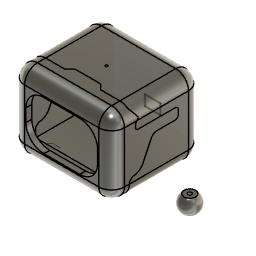
Astrobot clock outside v14 (Autodesk Fusion 360 design; units mm, degrees)
Autodesk Fusion 360 part; units mm, degrees
sketch "Sketch2" plane through (0, 0, 0) normal (0, 0, 1) x (1, 0, 0)
  line L0 (39, 35) -> (-39, 35)
  line L1 (-39, 35) -> (-39, -35)
  line L2 (-39, -35) -> (39, -35)
  line L3 (39, -35) -> (39, 35)
  line L4 (39, 35) -> (-39, -35) construction
  line L5 (-39, 35) -> (39, -35) construction
  dimension "d5" = 78
  dimension "d6" = 70
  constraint horizontal L0
  constraint perpendicular L0 L1
  constraint parallel L0 L2
  constraint parallel L1 L3
  constraint coincident L4 origin
  constraint coincident L5 origin
  measures "d5" distance of L1.end L2.end
  measures "d6" distance of L0.end L1.end
extrude "Extrude1" add sketch "Sketch2" along normal blind 60 makes body 1
fillet "Fillet2" radius 10 10 edges at (-39, 35, 30) (39, -35, 30) (0, 35, 0) (0, -35, 60) (39, 35, 30) (39, 0, 0) (-39, -35, 30) (-39, 0, 60) (-39, 0, 0) (39, 0, 60) 5 faces at (39, -11.6667, 20) (-39, 11.6667, 20) (-13, -35, 40) (13, -11.6667, 0) (13, 35, 40) on bodies 1
sketch "Sketch19" plane through (0, -35, 0) normal (0, -1, 0) x (1, 0, 0)
  line L0 (-29, 10) -> (29, 10)
  line L1 (29, 10) -> (29, 50)
  line L2 (29, 50) -> (-29, 50)
  line L3 (-29, 50) -> (-29, 10)
  line L4 (-14, 50) -> (14, 50)
  line L5 (29, 35) -> (29, 25)
  line L6 (14, 10) -> (-14, 10)
  line L7 (-29, 25) -> (-29, 35)
  arc A0 (-14, 50) -> (-29, 35) centre (-14, 35) ccw
  arc A1 (-29, 25) -> (-14, 10) centre (-14, 25) ccw
  arc A2 (14, 10) -> (29, 25) centre (14, 25) ccw
  arc A3 (29, 35) -> (14, 50) centre (14, 35) ccw
  arc A4 (28, 35) -> (14, 49) centre (14, 35) ccw
  line L8 (-14, 49) -> (14, 49)
  arc A5 (-14, 49) -> (-28, 35) centre (-14, 35) ccw
  line L9 (-28, 25) -> (-28, 35)
  arc A6 (-28, 25) -> (-14, 11) centre (-14, 25) ccw
  line L10 (14, 11) -> (-14, 11)
  arc A7 (14, 11) -> (28, 25) centre (14, 25) ccw
  line L11 (28, 35) -> (28, 25)
  dimension "d109" = 15
  dimension "d110" = 1
  constraint horizontal L4
  constraint vertical L5
  constraint horizontal L6
  constraint vertical L7
  constraint tangent L4 A0
  constraint tangent L7 A0
  constraint tangent L6 A1
  constraint tangent L7 A1
  constraint equal A0 A1
  constraint tangent L5 A2
  constraint tangent L6 A2
  constraint equal A0 A2
  constraint tangent L4 A3
  constraint tangent L5 A3
  constraint equal A0 A3
  measures "d109" radius of A0
extrude "Extrude15" cut sketch "Sketch19" against normal blind 42 contours A4 L8 A5 L9 A6 L10 A7 L11 bodies 1
sketch "Sketch3" plane through (39, 0, 0) normal (1, 0, 0) x (0, 1, 0)
  line L0 (-25, 10) -> (25, 10)
  line L1 (25, 10) -> (25, 50)
  line L2 (25, 50) -> (-25, 50)
  line L3 (-25, 50) -> (-25, 10)
  line L4 (-18.6068, 75) -> (-18.6068, 57.9889)
  line L5 (-18.6068, 57.9889) -> (-13.9508, 51.5222)
  line L6 (-13.9508, 51.5222) -> (-16.313, 48.3417)
  line L7 (-15.1681, 43.7622) -> (14.5844, 43.7622)
  line L8 (17.1014, 43.7622) -> (17.1014, 42.6668)
  line L9 (14.5617, 35.4315) -> (0.4578, 35.4315)
  line L10 (-4.0631, 32.5672) -> (-10, 20)
  arc A0 (-18.7241, 13.8606) -> (-10, 20) centre (-18.605, 22.9596) ccw
  line L11 (-21.0542, 11.5608) -> (-21.0542, 0)
  line L12 (-21.0542, 0) -> (-21.0542, -15)
  line L13 (-21.0542, -15) -> (-21.0542, -16.3731)
  spline S0 degree 5 poles (17.1014, 43.7622) (17.189, 43.7622) (17.3347, 43.7478) (17.4648, 43.6829) (17.4892, 43.5233) (17.3771, 43.252) (17.2511, 43.0139) (17.1681, 42.8378) (17.1221, 42.7233) (17.1014, 42.6668) knots 0 0 0 0 0 0 0.2 0.4 0.6 0.8 1 1 1 1 1 1
  line L14 (17.0843, 41.2452) -> (17.0617, 37.9145)
  arc A1 (17.0843, 41.2452) -> (14.5844, 43.7622) centre (14.5844, 41.2622) ccw
  arc A2 (14.5617, 35.4315) -> (17.0617, 37.9145) centre (14.5617, 37.9315) ccw
  arc A3 (0.4578, 35.4315) -> (-4.0631, 32.5672) centre (0.4578, 30.4315) ccw
  line L15 (-16.313, 48.3417) -> (-16.313, 44.9071)
  line L16 (-16.313, 44.9071) -> (-15.1681, 43.7622)
  line L17 (-18.7241, 13.8606) -> (-21.0542, 11.5608)
  point P0 (-16.313, 43.7622)
  dimension "d113" = 2.5
  dimension "d114" = 5
  dimension "d116" = 1.1449
  dimension "d117" = 1.1449
  constraint vertical L4
  constraint horizontal L7
  constraint perpendicular L7 L8
  constraint parallel L7 L9
  constraint perpendicular L0 L11
  constraint perpendicular L0 L12
  constraint perpendicular L0 L13
  constraint coincident L8.start L7
  constraint coincident L8.start L14
  constraint tangent L7 A1
  constraint tangent L14 A1
  constraint tangent L14 A2
  constraint tangent L9 A2
  constraint equal A1 A2
  constraint tangent L9 A3
  constraint tangent L10 A3
  constraint perpendicular L7 L15
  constraint coincident L15 P0
  constraint coincident L7 P0
  measures "d113" radius of A1
  measures "d114" radius of A3
  measures "d116" distance of L15.end P0
  measures "d117" distance of L7.start P0
split "Split1" by curves path "Sketch3" along L4 L5 L6 L15 L16 L7 A1 L14 A2 L9 A3 L10 A0 L17 L11 L12 L13 bodies 1 makes body 2 at (-9.6667, 9.6486, 0)
sketch "Sketch6" plane through (0, 0, 0) normal (0, 0, 1) x (1, 0, 0)
  line L0 (34, 30) -> (-34, 30)
  line L1 (-34, 30) -> (-34, -30)
  line L2 (-34, -30) -> (34, -30)
  line L3 (34, -30) -> (34, 30)
  line L4 (34, 30) -> (-34, -30) construction
  line L5 (-34, 30) -> (34, -30) construction
  dimension "d13" = 68
  dimension "d14" = 60
  constraint horizontal L0
  constraint perpendicular L0 L1
  constraint parallel L0 L2
  constraint parallel L1 L3
  constraint coincident L4 origin
  constraint coincident L5 origin
  measures "d13" distance of L1.end L2.end
  measures "d14" distance of L0.end L1.end
extrude "Extrude3" add sketch "Sketch6" along normal blind 50 separate body makes body 3
move_face "OffsetFaces1" offset 0.4 6 faces at (-11.3333, -30, 16.6667) (-34, 10, 33.3333) (-11.3333, 10, 50) (-11.3333, 10, 0) (34, -10, 33.3333) (11.3333, 30, 16.6667) on bodies 3
move_body "Move1" bodies 3 to x (1, 0, 0) y (0, 1, 0) z (0, 0, 1) at (0, 0, 5)
sketch "Sketch9" plane through (0, 0, 60) normal (0, 0, 1) x (-1, 0, 0)
  line L0 (-29, -25) -> (29, -25)
  line L1 (29, -25) -> (29, 18.6068)
  circle A0 centre (0, 0) radius 0.9
  line L2 (-29, 18.6068) -> (-29, -25)
  line L3 (29, 18.6068) -> (-29, 18.6068)
  dimension "d17" = 1.8
  constraint coincident A0.centre origin
  measures "d17" diameter of A0
extrude "Extrude4" cut sketch "Sketch9" against normal blind 3 contours A0 bodies 2
combine "Combine18" operation cut target body 2 tool bodies 3 keep tools
combine "Combine20" operation cut target body 1 tool bodies 3 keep tools
sketch "Sketch15" plane through (0, -18.6068, 0) normal (0, 1, 0) x (-1, 0, 0)
  arc A0 (-29, 60) -> (-35.0148, 57.9889) centre (-29, 50) ccw
  line L0 (-35.0148, 57.9889) -> (35.0148, 57.9889)
  arc A1 (35.0148, 57.9889) -> (29, 60) centre (29, 50) ccw
  line L1 (29, 60) -> (-29, 60)
  line L2 (10, 55.9778) -> (-10, 55.9778)
  line L3 (-10, 55.9778) -> (-10, 60)
  line L4 (-10, 60) -> (10, 60)
  line L5 (10, 60) -> (10, 55.9778)
  line L6 (10, 55.9778) -> (-10, 60) construction
  line L7 (-10, 55.9778) -> (10, 60) construction
  point P0 (0, 57.9889)
  constraint horizontal L2
  constraint perpendicular L2 L3
  constraint parallel L2 L4
  constraint parallel L3 L5
  constraint coincident L6 P0
  constraint coincident L7 P0
  constraint midpoint L0 P0
  constraint coincident L1 L3.end
extrude "Extrude11" add sketch "Sketch15" along normal blind 4 contours L0 L1 L3 L4 L5 bodies 1
chamfer "Chamfer1" distance 4 angle 45 2 edges at (10, -18.6068, 58.9944) (-10, -18.6068, 58.9944) on bodies 1
sketch "Sketch16" plane through (0, -21.0542, 0) normal (0, 1, 0) x (-1, 0, 0)
  line L0 (34.4, 11.5608) -> (34.4, 4.6)
  line L1 (34.4, 4.6) -> (-34.4, 4.6)
  line L2 (-34.4, 4.6) -> (-34.4, 11.5608)
  line L3 (-39, 11.5608) -> (-39, 10)
  arc A0 (-39, 10) -> (-29, 0) centre (-29, 10) ccw
  line L4 (-29, 0) -> (29, 0)
  arc A1 (29, 0) -> (39, 10) centre (29, 10) ccw
  line L5 (39, 10) -> (39, 11.5608)
  line L6 (-24, 4) -> (-18, 4)
  line L7 (-18, 4) -> (-18, 1)
  line L8 (-18, 1) -> (-24, 1)
  line L9 (-24, 1) -> (-24, 4)
  line L10 (0, 20) -> (0, 2.5)
  line L11 (18, 1) -> (24, 1)
  line L12 (24, 1) -> (24, 4)
  line L13 (18, 4) -> (18, 1)
  line L14 (24, 4) -> (18, 4)
  line L15 (-34.4, 11.5608) -> (-39, 11.5608)
  line L16 (39, 11.5608) -> (34.4, 11.5608)
  constraint horizontal L6
  constraint vertical L7
  constraint horizontal L8
  constraint vertical L9
  constraint symmetric L6.start L10 L12.end
  constraint symmetric L6.end L10 L13.start
  constraint symmetric L7.end L10 L11.start
  constraint symmetric L8.end L10 L11.end
extrude "Extrude12" add sketch "Sketch16" along normal blind 3 contours L6 L7 L8 L9 | L11 L12 L13 L14 bodies 1
chamfer "Chamfer2" distance 3 angle 45 4 edges at (18, -21.0542, 2.5) (-24, -21.0542, 2.5) (-18, -21.0542, 2.5) (24, -21.0542, 2.5) on bodies 1
combine "Combine21" operation cut target body 2 tool bodies 1 keep tools
split "Split3" by plane through (0, 0, 0) normal (1, 0, 0) bodies 1 makes body 4 at (34.4, -21.8123, 38.0559)
sketch "Sketch17" plane through (0, 35, 0) normal (0, 1, 0) x (-1, 0, 0)
  line L0 (-29, 10) -> (29, 10)
  line L1 (29, 10) -> (29, 50)
  line L2 (29, 50) -> (-29, 50)
  line L3 (-29, 50) -> (-29, 10)
  line L4 (-7, 20.6) -> (5, 20.6)
  line L5 (5, 20.6) -> (5, 12.6)
  line L6 (5, 12.6) -> (-7, 12.6)
  line L7 (-7, 12.6) -> (-7, 20.6)
  dimension "d91" = 12
  dimension "d92" = 8
  dimension "d93" = 22
  dimension "d94" = 2.6
  constraint horizontal L4
  constraint vertical L5
  constraint horizontal L6
  constraint vertical L7
  measures "d91" distance of L4.start L4.end
  measures "d92" distance of L4.start L6.end
  measures "d93" distance of L3 L4.start
  measures "d94" distance of L0 L6
extrude "Extrude14" cut sketch "Sketch17" against normal blind 8 contours L4 L5 L6 L7 bodies 2
sphere "SpherePrimitive1" add diameter 15 placed x (0, 1, 0) y (0, 0, 1) z (1, 0, 0) at (0, 0, 0) separate body makes body 5
ref_plane "WorkPlane1" through (0, 0, 7) normal (0, 0, 1) x (1, 0, 0)
split "Split4" by plane through (0, 0, 7) normal (0, 0, 1) bodies 5 makes body 6 at (0.4574, -0.6863, 7.4545)
hole "Hole2" at (0, 0, 7) direction (0, 0, -1) diameter 3 depth 10 tip angle 118 counterbore diameter 22 counterbore depth 1 bodies 5
combine "Combine22" operation add target body 4 tool bodies 1 keep tools
move_body "Move2" bodies 5 to x (1, 0, 0) y (0, 1, 0) z (0, 0, 1) at (65, 0, 0)
hidden bodies 1 3 6
equation "d117 = d116"
named bodies: "white", "inside", "blue", "white (1)"
